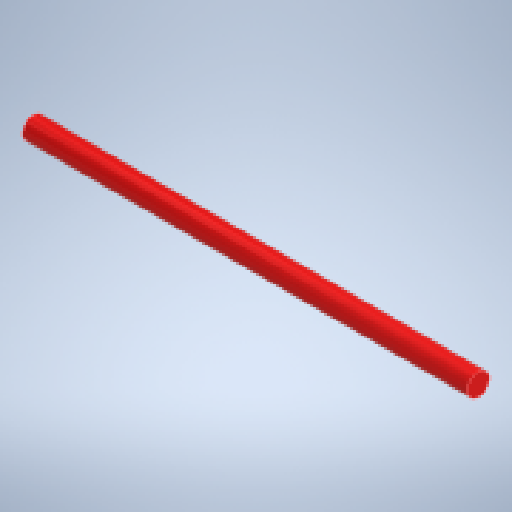
# Autodesk Inventor part: cable
Saved by Autodesk Inventor 2025.2 (Build 292293000, 293)
## iProperties
Created: 2025-06-25
Part Number: cable
Material: 一般
Document SubType Name: Modeling
Designer: naka6
Density: 1 g/cm^3
Appearance: 滑らか - 赤
Author: naka6
Autodesk Inventor part; units mm, degrees
ref_plane "YZ Plane" through (0, 0, 0) normal (1, 0, 0) x (0, 1, 0)
ref_plane "XZ Plane" through (0, 0, 0) normal (0, 1, 0) x (-1, 0, 0)
ref_plane "XY Plane" through (0, 0, 0) normal (0, 0, 1) x (1, 0, 0)
sketch "スケッチ1" plane through (0, 0, 0) normal (1, 0, 0) x (0, 1, 0)
  circle A0 centre (0, 0) radius 0.25
  dimension "d0" = 0.5
  constraints: 1 centre point, 1 coincident
  measures "d0" diameter of A0
extrude "押し出し1" add sketch "スケッチ1" along normal blind 1
sketch "スケッチ2" plane through (1, 0, 0) normal (1, 0, 0) x (0, 0, -1)
  circle A0 centre (0, 0) radius 0.25
  line L0 (3, -0.6634) -> (3, 0.6005)
  point P0 (3, 0)
  dimension "d3" = 3
  constraints: 2 end point, 1 centre point, 1 coincident, 1 point on line, 1 vertical
  measures "d3" distance of point (0, 0) point (3, 0)
revolve "回転1" add sketch "スケッチ2" angle 100 about axis through (1, -0.6634, -3) along (0, 1, 0)
sketch "スケッチ3" plane through (3.9544, 0, -3.5209) normal (-0.1736482, 0, -0.9848078) x (-0.9848078, 0, 0.1736482)
  circle A0 centre (0, 0) radius 0.25 projected
  point P0 (4.5058, 0)
extrude "押し出し2" add sketch "スケッチ3" along normal blind 22.5
sketch "スケッチ4" plane through (0.0473, 0, -25.6791) normal (-0.1736482, 0, -0.9848078) x (-0.9848078, 0, 0.1736482)
  circle A0 centre (0, 0) radius 0.25 projected
  line L0 (-2, -0.6001) -> (-2, 0.5446)
  point P0 (4.5058, 0)
  point P1 (-2, 0)
  dimension "d7" = 2
  constraints: 2 end point, 1 point on line, 1 vertical
  measures "d7" distance of A0.centre point (-2, 0)
revolve "回転2" add sketch "スケッチ4" angle 100 about axis through (2.017, -0.6001, -26.0264) along (0, -1, 0)
